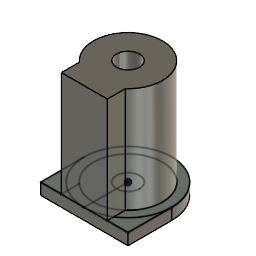
hexbug_station_cap (Autodesk Fusion 360 design; units mm, degrees)
Autodesk Fusion 360 part; units mm, degrees
note: some values were not read from the file. Set by a fixed rule: which sketch regions a step uses.
sketch "Sketch1" plane through (0, 0, 0) normal (0, 0, 1) x (1, 0, 0)
  circle A0 centre (0, 0) radius 3.75
  circle A1 centre (0, 0) radius 1.25
  circle A2 centre (0, 0) radius 4.75
  line L0 (0, 0) -> (0, -4.75)
  line L1 (0, -4.75) -> (2.5, -4.75)
  line L2 (0, -4.75) -> (-2.5, -4.75)
  line L3 (2.5, -4.75) -> (2.5, -2.7951)
  line L4 (-2.5, -4.75) -> (-2.5, -2.7951)
  line L5 (2.5, -4.75) -> (4.75, -4.75)
  line L6 (4.75, -4.75) -> (4.75, 0)
  line L7 (-4.75, 0) -> (-4.75, -4.75)
  line L8 (-4.75, -4.75) -> (-2.5, -4.75)
  dimension "d1" = 7.5
  dimension "d2" = 2.5
  dimension "d3" = 9.5
  dimension "d4" = 2.5
  dimension "d5" = 2.5
  dimension "d10" = 2.25
  constraint coincident A0.centre A1.centre
  constraint coincident A2 L0.end
  constraint vertical L0
  constraint perpendicular L0 L1
  constraint perpendicular L0 L2
  constraint coincident A0 L3.end
  constraint perpendicular L1 L3
  constraint coincident A0 L4.end
  constraint perpendicular L2 L4
  constraint perpendicular L3 L5
  constraint coincident A2 L6.end
  constraint tangent A2 L6
  constraint coincident A2 L7.start
  constraint tangent A2 L7
  constraint parallel L6 L7
  constraint perpendicular L4 L8
  measures "d1" diameter of A0
  measures "d2" diameter of A1
  measures "d3" diameter of A2
  measures "d4" distance of L0.end L1.end
  measures "d5" distance of L0.end L2.end
  measures "d10" distance of L1.end L5.end
extrude "Extrude1" add sketch "Sketch1" along normal blind 5 contours A0 | A0 A2 L0 L4 | A0 A2 L0 L3 | A2 L2 L4 | A2 L1 L3
extrude "Extrude2" add sketch "Sketch1" along normal blind 2 contours A1
extrude "Extrude3" add sketch "Sketch1" against normal blind 1.25 contours A0 | A0 A2 L3 L4 | A0 A2 L0 L4 | A0 A2 L0 L3 | A2 L4 L7 L8 | A2 L2 L4 | A2 L1 L3 | A2 L3 L5 L6 | A1
extrude "Extrude4" add 1 faces at (0.0311, -3.5822, 5) along direction (0, 0, 1) blind 6.444
extrude "Extrude5" [suppressed]
extrude "Extrude6" [suppressed]
